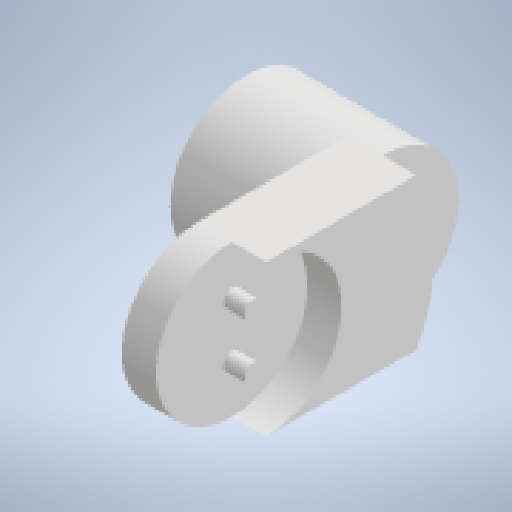
# Autodesk Inventor part: Herramienta Marcador Conector
Saved by Autodesk Inventor 2023 (Build 270158000, 158)
## iProperties
Created: 2023-02-19
Part Number: Herramienta Marcador Conector
Material: Generic
Document SubType Name: Modeling
Designer: luisd
Density: 1 g/cm^3
Appearance: Default
Author: luisd
Autodesk Inventor part; units mm, degrees
ref_plane "YZ Plane" through (0, 0, 0) normal (1, 0, 0) x (0, 1, 0)
ref_plane "XZ Plane" through (0, 0, 0) normal (0, 1, 0) x (-1, 0, 0)
ref_plane "XY Plane" through (0, 0, 0) normal (0, 0, 1) x (1, 0, 0)
sketch "Sketch1" plane through (0, 0, 0) normal (1, 0, 0) x (0, 1, 0)
  circle A0 centre (4.0001, 0) radius 1.25
  circle A1 centre (-3.9999, 0) radius 1.25
  circle A2 centre (0, 0) radius 11
  line L0 (11, 0) -> (11, -22)
  line L1 (11, 0) -> (33, 0) construction
  line L2 (-11, 0) -> (-11, -22)
  line L3 (-11, 0) -> (11, 0) construction
  circle A3 centre (0, -22) radius 11
  circle A4 centre (0, -26.0001) radius 1.25
  circle A5 centre (0, -18.0001) radius 1.25
  point P0 (1.5875, 1.5875)
  dimension "d0" = 22
  dimension "d1" = 90
  dimension "d2" = 22
  dimension "d3" = 90
  constraints: 8 end point, 5 centre point, 2 horizontal, 2 perpendicular, 2 point on circle, 2 vertical, 1 tangent, 3 other
  measures "d0" distance of L0.start L0.end
  measures "d1" angle of L0 L1
  measures "d2" distance of L2.start L2.end
  measures "d3" angle of L2 L3
extrude "Extrusion1" add sketch "Sketch1" along normal blind 5
sketch "Sketch2" plane through (5, 0, 0) normal (1, 0, 0) x (0, 0, -1)
  arc A0 (0, 11) -> (0, -11) centre (0, 0) ccw projected
  line L0 (0, -11) -> (22, -11) projected
  arc A1 (22, -11) -> (22, 11) centre (22, 0) ccw projected
  line L1 (22, 11) -> (0, 11) projected
  circle A2 centre (18.0001, 0) radius 1.25 projected
  circle A3 centre (26.0001, 0) radius 1.25 projected
  circle A4 centre (0, -3.9999) radius 1.25 projected
  circle A5 centre (0, 4.0001) radius 1.25 projected
extrude "Extrusion2" add sketch "Sketch2" along normal blind 3 and the other way blind 5 contours A4 | A5
sketch "Sketch3" plane through (0, 0, 0) normal (-1, 0, 0) x (0, 0, 1)
  arc A0 (0, -11) -> (0, 11) centre (0, 0) ccw projected
  line L0 (0, -11) -> (-22, -11) projected
  arc A1 (-22, 11) -> (-22, -11) centre (-22, 0) ccw projected
  line L1 (-22, 11) -> (0, 11) projected
  circle A2 centre (-18.0001, 0) radius 1.25 projected
  circle A3 centre (-26.0001, 0) radius 1.25 projected
  circle A4 centre (0, -3.9999) radius 1.25 projected
  circle A5 centre (0, 4.0001) radius 1.25 projected
extrude "Extrusion3" add sketch "Sketch3" against normal blind 5 contours A2 | A3
sketch "Sketch4" plane through (0, 0, 0) normal (-1, 0, 0) x (0, 0, 1)
  line L0 (0, 0) -> (-22, 0)
  line L1 (0, 0) -> (22, 0) construction
  circle A0 centre (-22, 0) radius 11
  circle A1 centre (-22, 0) radius 9.5
  dimension "d12" = 22
  dimension "d13" = 180
  dimension "d14" = 22
  dimension "d15" = 19
  constraints: 4 end point, 2 centre point, 2 coincident, 2 horizontal, 1 collinear
  measures "d12" distance of L0.start L0.end
  measures "d13" angle of L0 L1
  measures "d14" diameter of A0
  measures "d15" diameter of A1
extrude "Extrusion4" add sketch "Sketch4" along normal blind 15 contours A1 | A0
sketch "Sketch5" plane through (5, 0, 0) normal (1, 0, 0) x (0, 0, -1)
  circle A0 centre (0, 0) radius 24.5 projected
  circle A1 centre (-20, 0) radius 3.5 projected
  circle A2 centre (-14.1421, 14.1421) radius 2.675 projected
  circle A3 centre (-14.1421, -14.1421) radius 2.675 projected
  circle A4 centre (14.1421, -14.1421) radius 2.675 projected
  circle A5 centre (14.1421, 14.1421) radius 2.675 projected
  circle A6 centre (0, 0) radius 11 projected
  line L0 (0, -11) -> (22, -11) projected
  line L1 (22, 11) -> (0, 11) projected
  point P0 (0, 0)
  point P1 (21.8918, 11)
  point P2 (21.8918, -11)
extrude "Extrusion5" add sketch "Sketch5" along normal blind 5 contours A0 L0 A6 L1 picked at (19.9018, -1.2624)
sketch "Sketch6" plane through (-15, 0, -22) normal (-1, 0, 0) x (0, 0, 1)
  circle A0 centre (0, 0) radius 7.5
  point P0 (22, 0)
  dimension "d20" = 15
  constraints: 1 centre point
  measures "d20" diameter of A0
extrude "Extrusion6" cut sketch "Sketch6" against normal blind 15
body "Solid1"
